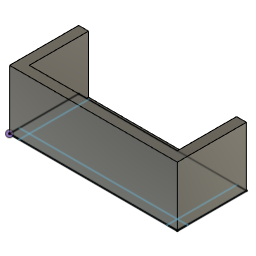
Arm (Autodesk Fusion 360 design; units mm, degrees)
Autodesk Fusion 360 part; units mm, degrees
sketch "Sketch1" plane through (0, 0, 0) normal (0, 0, 1) x (1, 0, 0)
  line L0 (0, 0) -> (170, 0)
  line L1 (170, 0) -> (170, 70)
  line L2 (170, 70) -> (0, 70)
  line L3 (0, 70) -> (0, 0)
  line L4 (0, 70) -> (10, 70)
  line L5 (10, 70) -> (10, 0)
  line L6 (10, 0) -> (0, 0)
  line L7 (0, 0) -> (0, 70)
  line L8 (0, 10) -> (170, 10)
  line L9 (170, 10) -> (170, 0)
  line L10 (170, 0) -> (0, 0)
  line L11 (0, 0) -> (0, 10)
  line L12 (170, 0) -> (160, 0)
  line L13 (160, 0) -> (160, 70)
  line L14 (160, 70) -> (170, 70)
  line L15 (170, 70) -> (170, 0)
  dimension "d1" = 170
  dimension "d2" = 70
  constraint horizontal L0
  constraint vertical L1
  constraint horizontal L2
  constraint vertical L3
  constraint coincident L0.start L3.end
  constraint horizontal L4
  constraint vertical L5
  constraint horizontal L6
  constraint vertical L7
  constraint coincident L0 L5.end
  constraint horizontal L8
  constraint vertical L9
  constraint horizontal L10
  constraint vertical L11
  constraint coincident L3 L8.start
  constraint horizontal L12
  constraint vertical L13
  constraint horizontal L14
  constraint vertical L15
  constraint coincident L2 L13.end
  measures "d1" distance of L0.start L0.end
  measures "d2" distance of L0.start L2.end
extrude "Extrude1" add sketch "Sketch1" along normal blind 2 contours L2 L5 L8 L13
extrude "Extrude2" add sketch "Sketch1" along normal blind 60 contours L0 L3 L5 L6 L7 L8 L10 L11 | L0 L5 L8 L10 L13 | L2 L3 L4 L5 L7 L8 | L0 L1 L8 L9 L10 L12 L13 L15 | L1 L2 L8 L13 L14 L15
